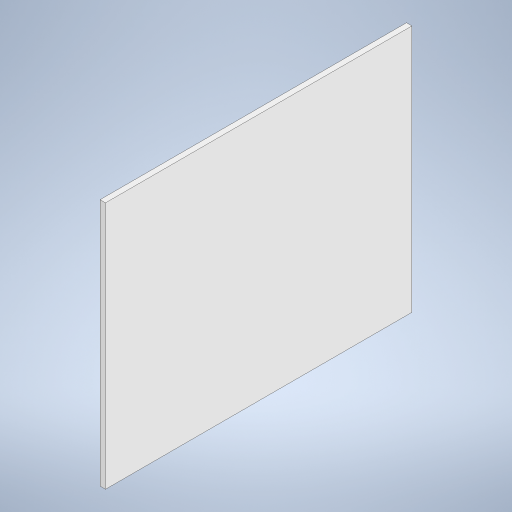
# Autodesk Inventor part: Plywood--0.75_x_34_x_42.75_in
Saved by Autodesk Inventor 2024 (Build 280153000, 153)
## iProperties
Created: 2023-05-06
Part Number: Plywood--0.75_x_34_x_42.75_in
Material: Generic
Document SubType Name: Modeling
Designer: Tom
Density: 1 g/cm^3
Appearance: White
Author: Tom
Autodesk Inventor part; units mm, degrees
ref_plane "YZ Plane" through (0, 0, 0) normal (1, 0, 0) x (0, 1, 0)
ref_plane "XZ Plane" through (0, 0, 0) normal (0, 1, 0) x (-1, 0, 0)
ref_plane "XY Plane" through (0, 0, 0) normal (0, 0, 1) x (1, 0, 0)
sketch "Sketch1" plane through (0, 0, 0) normal (1, 0, 0) x (0, 1, 0)
  line L0 (0, 0) -> (863.6, 0)
  line L1 (863.6, 0) -> (863.6, -1066.8)
  line L2 (863.6, -1066.8) -> (0, -1066.8)
  line L3 (0, -1066.8) -> (0, 0)
  dimension "d1" = 1066.8
  dimension "d2" = 863.6
  constraints: 8 end point, 2 parallel, 1 horizontal, 1 perpendicular
  measures "d1" distance of L0.end L1.end
  measures "d2" distance of L1.end L2.end
extrude "Extrusion1" add sketch "Sketch1" along normal blind 19.05
body "Solid1"
